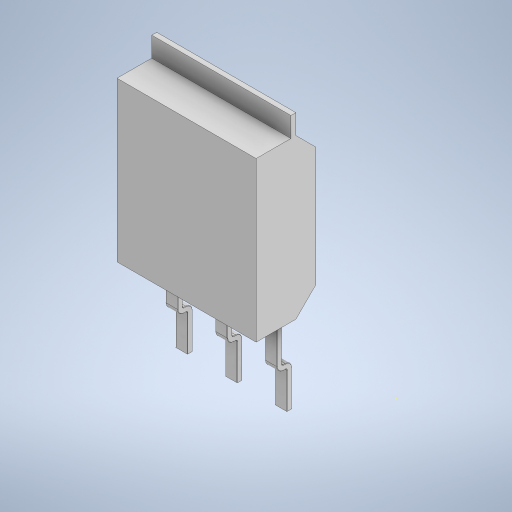
# Autodesk Inventor part: LM7805
Saved by Autodesk Inventor 2024 (Build 280153000, 153)
## iProperties
Created: 2023-12-15
Part Number: LM7805
Material: Generic
Document SubType Name: Sheet Metal
Designer: user
Density: 1 g/cm^3
Sheet Metal Rule: Default
Appearance: Default
Author: user
Autodesk Inventor part; units mm, degrees
sketch "Sketch1" plane through (0, 0, 0) normal (0, 0, 1) x (1, 0, 0)
  line L0 (-11.0258, 9.9444) -> (-4.0258, 9.9444)
  line L1 (-4.0258, 9.9444) -> (-4.0258, 1.9444)
  line L2 (-4.0258, 1.9444) -> (-11.0258, 1.9444)
  line L3 (-11.0258, 1.9444) -> (-11.0258, 9.9444)
  point P0 (0, 0)
  dimension "d0" = 7
  dimension "d1" = 8
  constraints: 8 end point, 2 parallel, 1 horizontal, 1 perpendicular
  measures "d0" distance of L1.end L2.end
  measures "d1" distance of L0.end L1.end
extrude "Extrusion1" add sketch "Sketch1" along normal mid plane 3
chamfer "Chamfer1" distance 1 angle 45 2 edges at (-7.5258, 9.9444, -1.5) (-7.5258, 1.9444, -1.5)
sketch "Sketch2" plane through (-11.0258, 1.9444, 1.5) normal (0, -1, 0) x (1, 0, 0)
  line L0 (0, 0) -> (7, 0) projected
  line L1 (1.28, -2) -> (1, -2)
  line L2 (5.72, -2) -> (6, -2)
  line L3 (3.78, -1.75) -> (3.22, -1.75)
  line L4 (3.2, -1.77) -> (3.2, -1.98)
  line L5 (3.22, -2) -> (3.78, -2)
  line L6 (3.8, -1.98) -> (3.8, -1.77)
  line L7 (6, -2) -> (6, -1.75)
  line L8 (6, -1.75) -> (6.3, -1.75)
  line L9 (1, -1.75) -> (0.72, -1.75)
  line L10 (1.3, -1.77) -> (1.3, -1.98)
  line L11 (0.7, -1.98) -> (0.7, -1.77)
  line L12 (6.28, -1.75) -> (5.72, -1.75)
  line L13 (5.7, -1.77) -> (5.7, -1.98)
  line L14 (5.7, -2) -> (6.28, -2)
  line L15 (6.3, -1.98) -> (6.3, -1.77)
  line L16 (2.1489, -1.875) -> (2.3953, -1.875)
  line L17 (1, -0.9318) -> (1, -0.5966)
  line L18 (3.5, -0.8962) -> (3.5, -0.5966)
  line L19 (6, -1.2102) -> (6, -1.0883)
  arc A0 (6.3, -1.77) -> (6.28, -1.75) centre (6.28, -1.77) ccw
  arc A1 (5.72, -1.75) -> (5.7, -1.77) centre (5.72, -1.77) ccw
  arc A2 (5.7, -1.98) -> (5.72, -2) centre (5.72, -1.98) ccw
  arc A3 (6.28, -2) -> (6.3, -1.98) centre (6.28, -1.98) ccw
  arc A4 (3.8, -1.77) -> (3.78, -1.75) centre (3.78, -1.77) ccw
  arc A5 (3.22, -1.75) -> (3.2, -1.77) centre (3.22, -1.77) ccw
  arc A6 (3.2, -1.98) -> (3.22, -2) centre (3.22, -1.98) ccw
  arc A7 (3.78, -2) -> (3.8, -1.98) centre (3.78, -1.98) ccw
  arc A8 (1.3, -1.77) -> (1.28, -1.75) centre (1.28, -1.77) ccw
  arc A9 (0.72, -1.75) -> (0.7, -1.77) centre (0.72, -1.77) ccw
  arc A10 (0.7, -1.98) -> (0.72, -2) centre (0.72, -1.98) ccw
  arc A11 (1.28, -2) -> (1.3, -1.98) centre (1.28, -1.98) ccw
  line L20 (0.72, -2) -> (1, -2)
  line L21 (1.28, -1.75) -> (1, -1.75)
  point P0 (11.0258, -1.5)
  point P1 (3.5, -2)
  point P2 (3.2, -2)
  point P3 (3.8, -2)
  point P4 (0.7, -2)
  point P5 (6.3, -2)
  dimension "d7" = 2.5
  dimension "d8" = 2.5
  dimension "d13" = 0.6
  dimension "d14" = 0.25
  dimension "d15" = 0.3
  dimension "d16" = 0.25
  dimension "d19" = 0.6
  dimension "d31" = 0.02
  constraints: 42 end point, 24 point on circle, 22 tangent, 14 point on line, 12 centre point, 11 equal radius, 5 parallel, 4 horizontal, 3 perpendicular, 1 vertical
  measures "d7" distance of point (3.5, -2) L1.end
  measures "d8" distance of point (3.5, -2) L2.end
  measures "d13" distance of point (3.8, -2) point (3.2, -2)
  measures "d14" distance of L2.end L7.end
  measures "d15" distance of L7.end L8.end
  measures "d16" distance of L1.end L9.start
  measures "d19" distance of point (6.3, -2) L14.start
  measures "d31" radius of A0
sketch "Sketch3" plane through (-11.0258, 9.9444, 1.5) normal (0, 1, 0) x (1, 0, 0)
  line L0 (0, 2) -> (0, 0) projected
  line L1 (7, 2) -> (7, 0) projected
  line L2 (0, 2) -> (7, 2)
  line L3 (7, 2) -> (7, 1.75)
  line L4 (7, 1.75) -> (0, 1.75)
  line L5 (0, 1.75) -> (0, 2)
  point P0 (11.0258, 1.5)
  dimension "d20" = 0.25
  constraints: 8 end point, 2 parallel, 1 horizontal, 1 perpendicular, 1 point on line
  measures "d20" distance of L2.end L3.end
extrude "Extrusion2" add sketch "Sketch3" along normal blind 1
ref_plane "Work Plane1" through (-5.0258, 1.9444, 0.2898) normal (1, 0, 0) x (0, 0, 1)
ref_plane "Work Plane2" through (-7.5258, 1.9444, 0.6038) normal (1, 0, 0) x (0, 0, 1)
ref_plane "Work Plane3" through (-10.0258, 1.9444, 0.5682) normal (1, 0, 0) x (0, 0, 1)
sketch "Sketch4" plane through (-5.0258, 1.9444, 0.2898) normal (1, 0, 0) x (0, 0, 1)
  line L0 (-0.6648, 0) -> (-0.6648, 2.3)
  line L1 (-0.8648, 2.5) -> (-0.9648, 2.5)
  line L2 (-1.1648, 2.7) -> (-1.1648, 4.5)
  arc A0 (-0.6648, 2.3) -> (-0.8648, 2.5) centre (-0.8648, 2.3) ccw
  arc A1 (-1.1648, 2.7) -> (-0.9648, 2.5) centre (-0.9648, 2.7) ccw
  point P0 (-0.2898, 1.9444)
  point P1 (-0.7898, 0)
  point P2 (-0.6648, 2.5)
  point P3 (-1.1648, 2.5)
  dimension "d26" = 0.125
  dimension "d27" = 2.5
  dimension "d28" = 0.5
  dimension "d29" = 2
  dimension "d30" = 0.2
  constraints: 6 end point, 4 point on circle, 4 point on line, 4 tangent, 2 centre point, 2 perpendicular, 1 equal radius
  measures "d26" distance of point (-0.79, 0) L0.start
  measures "d27" distance of L0.start point (-0.665, 2.5)
  measures "d28" distance of point (-0.665, 2.5) point (-1.165, 2.5)
  measures "d29" distance of point (-1.165, 2.5) L2.end
  measures "d30" radius of A0
sweep "Sweep1" add profiles "Sketch2" path "Sketch4" contours A2 L13 A1 L12 L7 L2 | L7 L8 A0 L15 A3 L14
sketch "Sketch8" plane through (-7.5258, 1.9444, 0.6038) normal (1, 0, 0) x (0, 0, 1)
  line L0 (-0.9788, 0) -> (-0.9788, 2.3)
  line L1 (-1.1788, 2.5) -> (-1.2788, 2.5)
  line L2 (-1.4788, 2.7) -> (-1.4788, 4.5)
  arc A0 (-0.9788, 2.3) -> (-1.1788, 2.5) centre (-1.1788, 2.3) ccw
  arc A1 (-1.4788, 2.7) -> (-1.2788, 2.5) centre (-1.2788, 2.7) ccw
  point P0 (-0.6038, 1.9444)
  point P1 (-1.1038, 0)
  point P2 (-0.9788, 2.5)
  point P3 (-1.4788, 2.5)
  dimension "d55" = 0.125
  dimension "d56" = 2.5
  dimension "d57" = 0.5
  dimension "d58" = 2
  dimension "d59" = 0.2
  constraints: 6 end point, 4 point on circle, 4 point on line, 4 tangent, 2 centre point, 2 perpendicular, 1 equal radius
  measures "d55" distance of point (-1.104, 0) L0.start
  measures "d56" distance of L0.start point (-0.979, 2.5)
  measures "d57" distance of point (-0.979, 2.5) point (-1.479, 2.5)
  measures "d58" distance of point (-1.479, 2.5) L2.end
  measures "d59" radius of A0
sweep "Sweep2" add profiles "Sketch2" path "Sketch8" contours A4 L6 A7 L5 A6 L4 A5 L3
sketch "Sketch9" plane through (-10.0258, 1.9444, 0.5682) normal (1, 0, 0) x (0, 0, 1)
  line L0 (-0.9432, 0) -> (-0.9432, 2.3)
  line L1 (-1.1432, 2.5) -> (-1.2432, 2.5)
  line L2 (-1.4432, 2.7) -> (-1.4432, 4.5)
  arc A0 (-0.9432, 2.3) -> (-1.1432, 2.5) centre (-1.1432, 2.3) ccw
  arc A1 (-1.4432, 2.7) -> (-1.2432, 2.5) centre (-1.2432, 2.7) ccw
  point P0 (-0.5682, 1.9444)
  point P1 (-1.0682, 0)
  point P2 (-0.9432, 2.5)
  point P3 (-1.4432, 2.5)
  dimension "d62" = 0.125
  dimension "d63" = 2.5
  dimension "d64" = 0.5
  dimension "d65" = 2
  dimension "d66" = 0.2
  constraints: 6 end point, 4 point on circle, 4 point on line, 4 tangent, 2 centre point, 2 perpendicular, 1 equal radius
  measures "d62" distance of point (-1.068, 0) L0.start
  measures "d63" distance of L0.start point (-0.943, 2.5)
  measures "d64" distance of point (-0.943, 2.5) point (-1.443, 2.5)
  measures "d65" distance of point (-1.443, 2.5) L2.end
  measures "d66" radius of A0
sweep "Sweep3" add profiles "Sketch2" path "Sketch9" contours L1 L20 A10 L11 A9 L9 L21 A8 L10 A11
sketch "Sketch10" plane through (0, 0, -1.5) normal (0, 0, -1) x (-1, 0, 0)
  line L0 (3.9497, 6.7299) -> (11.068, 6.7299) construction
  line L1 (11.068, 6.7299) -> (11.068, 5.1619) construction
  line L2 (11.068, 5.1619) -> (3.9497, 5.1619) construction
  line L3 (3.9497, 5.1619) -> (3.9497, 6.7299) construction
  point P0 (0, 0)
  constraints: 2 other
equation "\"BendRadius\" = Thickness"
equation "\"BendReliefWidth\" = Thickness"
equation "\"BendReliefDepth\" = 0.5 * Thickness"
equation "\"CornerReliefSize\" = 4 * Thickness"
equation "\"MinimumRemnant\" = 2 * Thickness"
equation "\"TransitionRadius\" = BendRadius"
equation "\"JacobiRadiusSize\" = BendRadius"
equation "\"GapSize\" = Thickness"
equation "\"Thickness\" = 3.048"
body "Solid1"
